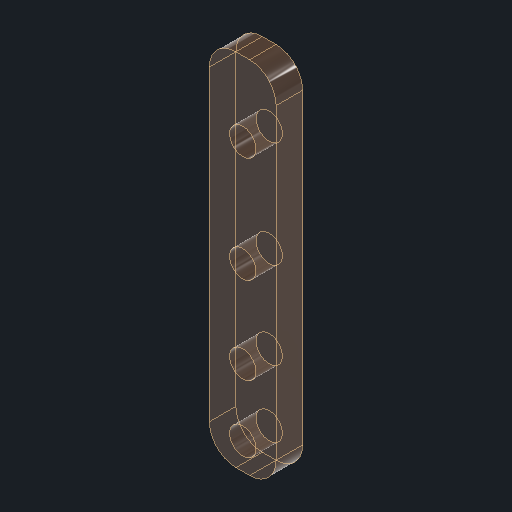
# Autodesk Inventor part: Claw7_Claw_Plate
Saved by Autodesk Inventor 2023 (Build 270158000, 158)
## iProperties
Created: 2023-12-30
Part Number: Claw7_Claw_Plate
Material: Polycarbonate, Smoke
Document SubType Name: Modeling
Designer: kelle
Density: 1.2 g/cm^3
Appearance: Polycarbonate - Smoked
Author: kelle
Autodesk Inventor part; units mm, degrees
ref_plane "YZ Plane" through (0, 0, 0) normal (1, 0, 0) x (0, 1, 0)
ref_plane "XZ Plane" through (0, 0, 0) normal (0, 1, 0) x (-1, 0, 0)
ref_plane "XY Plane" through (0, 0, 0) normal (0, 0, 1) x (1, 0, 0)
sketch "Sketch1" plane through (0, 0, 0) normal (0, 0, 1) x (1, 0, 0)
  line L0 (-4.0005, -21.59) -> (4.0005, -21.59)
  line L1 (4.0005, -21.59) -> (4.0005, 21.59)
  line L2 (4.0005, 21.59) -> (-4.0005, 21.59)
  line L3 (-4.0005, 21.59) -> (-4.0005, -21.59)
  line L4 (-4.0005, -21.59) -> (4.0005, 21.59) construction
  line L5 (4.0005, -21.59) -> (-4.0005, 21.59) construction
  circle A0 centre (0, -18.415) radius 1.5875
  circle A1 centre (0, -18.415) radius 2.1 construction
  circle A2 centre (0, -10.415) radius 1.5875
  circle A3 centre (0, 12.7) radius 1.5875
  circle A4 centre (0, 0) radius 1.5875
  dimension "d0" = 8.001
  dimension "d1" = 43.18
  dimension "d2" = 3.175
  dimension "d3" = 4.2
  dimension "d4" = 3.175
  dimension "d5" = 8
  dimension "d6" = 3.175
  dimension "d7" = 3.175
  dimension "d8" = 3.175
  dimension "d9" = 8.89
  dimension "d10" = 4.0005
  constraints: 12 end point, 5 centre point, 2 coincident, 2 midpoint, 2 parallel, 1 horizontal, 1 perpendicular
  measures "d0" distance of L2.end L1.end
  measures "d1" distance of L1.end L0.end
  measures "d2" diameter of A0
  measures "d3" diameter of A1
  measures "d4" diameter of A2
  measures "d5" distance of A0.centre A2.centre
  measures "d6" distance from line of L0 A0.centre
  measures "d7" diameter of A3
  measures "d8" diameter of A4
  measures "d9" distance from line of L2 A3.centre
  measures "d10" distance from line of L1 A3.centre
extrude "Extrusion1" add sketch "Sketch1" along normal blind 3.175
fillet "Fillet1" radius 3.175 4 edges at (-4.0005, 21.59, 1.5875) (4.0005, 21.59, 1.5875) (4.0005, -21.59, 1.5875) (-4.0005, -21.59, 1.5875)
body "Solid1"
